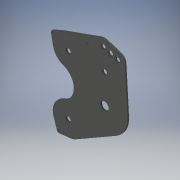
# Autodesk Inventor part: Shooter Side Plate
Saved by Autodesk Inventor 2019.4 (Build 234330000, 330)
## iProperties
Created: 2020-01-16
Part Number: Shooter Side Plate
Material: CFRP
Document SubType Name: Modeling
Designer: admin
Density: 1.43 g/cm^3
Appearance: Carbon Fiber
Mass: 572.525 g
Surface Area: 1689.26 cm^2
Volume: 400.367 cm^3
Author: admin
Autodesk Inventor part; units mm, degrees
ref_plane "YZ Plane" through (0, 0, 0) normal (1, 0, 0) x (0, 1, 0)
ref_plane "XZ Plane" through (0, 0, 0) normal (0, 1, 0) x (-1, 0, 0)
ref_plane "XY Plane" through (0, 0, 0) normal (0, 0, 1) x (1, 0, 0)
sketch "Sketch1" plane through (0, 0, 0) normal (0, 0, 1) x (1, 0, 0)
  arc A0 (88.7461, 5.2288) -> (44.314, -77.068) centre (0, 0) ccw construction
  circle A1 centre (0, 114.3) radius 50.8 construction
  circle A2 centre (-140.8057, 114.3) radius 50.8 construction
  circle A3 centre (-140.8057, -114.3) radius 50.8 construction
  line L0 (-140.8057, 114.3) -> (-140.8057, -114.3) construction
  line L1 (-140.8057, 0) -> (0, 0) construction
  circle A4 centre (-140.8057, -114.3) radius 9.5
  circle A5 centre (-140.8057, 114.3) radius 9.5
  circle A6 centre (0, 114.3) radius 9.5
  line L2 (0, 0) -> (0, 114.3) construction
  circle A7 centre (-4.9132, 197.2883) radius 9
  circle A8 centre (50.8994, 180.0301) radius 9
  line L3 (0, 114.3) -> (50.8994, 180.0301) construction
  line L4 (0, 114.3) -> (-4.9132, 197.2883) construction
  arc A9 (59.0234, 206.3028) -> (78.3518, 181.6476) centre (50.8994, 180.0301) ccw construction
  arc A10 (-14.1538, 223.1893) -> (3.2107, 223.561) centre (-4.9132, 197.2883) ccw construction
  line L5 (0, 0) -> (-490.9821, 0) construction
  line L6 (78.3518, 181.6476) -> (88.7461, 5.2288)
  line L7 (3.2107, 223.561) -> (59.0234, 206.3028)
  arc A11 (-160.967, 170.8112) -> (-160.2677, 57.5441) centre (-140.8057, 114.3) ccw
  arc A12 (-160.2677, -57.5441) -> (-110.8974, -166.3144) centre (-140.8057, -114.3) ccw
  line L8 (-160.967, 170.8112) -> (-14.1538, 223.1893)
  line L9 (-110.8974, -166.3144) -> (44.314, -77.068)
  arc A13 (-160.2677, -57.5441) -> (-160.2677, 57.5441) centre (-180, 0) ccw
  arc A14 (44.314, -77.068) -> (88.7461, 5.2288) centre (0, 0) ccw
  arc A15 (-160.2677, 57.5441) -> (-160.967, 170.8112) centre (-140.8057, 114.3) ccw construction
  arc A16 (-110.8974, -166.3144) -> (-160.2677, -57.5441) centre (-140.8057, -114.3) ccw construction
  circle A17 centre (0, 0) radius 16
  line L10 (-140.8057, -114.3) -> (0, 114.3) construction
  line L11 (-140.8057, 114.3) -> (-88.5835, 196.6353) construction
  circle A18 centre (22.9931, 188.6592) radius 22.86 construction
  circle A19 centre (-4.9132, 197.2883) radius 6.35 construction
  circle A20 centre (50.8994, 180.0301) radius 6.35 construction
  line L12 (-4.9132, 197.2883) -> (50.8994, 180.0301) construction
  arc A21 (3.2107, 223.561) -> (-14.1538, 223.1893) centre (-4.9132, 197.2883) ccw
  arc A22 (78.3518, 181.6476) -> (59.0234, 206.3028) centre (50.8994, 180.0301) ccw
  circle A23 centre (22.9931, 188.6592) radius 9.5
  line L13 (0, 114.3) -> (22.9931, 188.6592) construction
  line L14 (22.9931, 188.6592) -> (-140.8057, 114.3) construction
  circle A24 centre (-64.9132, 178.5367) radius 2.75
  circle A25 centre (64, 85.1942) radius 2.75
  dimension "d37" = 177.8
  dimension "d38" = 101.6
  dimension "d39" = 101.6
  dimension "d40" = 101.6
  dimension "d41" = 19
  dimension "d42" = 19
  dimension "d43" = 19
  dimension "d44" = 114.3
  dimension "d46" = 228.6
  dimension "d47" = 18
  dimension "d48" = 18
  dimension "d50" = 55
  dimension "d52" = 55
  dimension "d54" = 0
  dimension "d55" = 140.8057
  dimension "d58" = 120
  dimension "d59" = 120
  dimension "d60" = 180
  dimension "d61" = 32
  dimension "d64" = 268.485
  dimension "d67" = 97.5
  dimension "d77" = 45.72
  dimension "d78" = 12.7
  dimension "d79" = 12.7
  dimension "d80" = 19
  dimension "d81" = 77.833
  dimension "d82" = 179.887
  dimension "d90" = 5.5
  dimension "d91" = 25
  dimension "d92" = 60
  dimension "d93" = 5.5
  dimension "d94" = 20
  dimension "d95" = 64
  constraints: 30 end point, 26 centre point, 22 point on circle, 11 coincident, 11 tangent, 2 midpoint, 2 perpendicular, 2 point on line, 1 equal length, 1 horizontal
  measures "d37" diameter of A0
  measures "d38" diameter of A1
  measures "d39" diameter of A2
  measures "d40" diameter of A3
  measures "d41" diameter of A4
  measures "d42" diameter of A5
  measures "d43" diameter of A6
  measures "d44" distance of L1.end L2.end
  measures "d46" distance of L0.start L0.end
  measures "d47" diameter of A7
  measures "d48" diameter of A8
  measures "d50" diameter of A9
  measures "d52" diameter of A10
  measures "d54" distance between parallel lines of L1 L5
  measures "d55" distance from line of point (0, 0) L0
  measures "d58" diameter of A11
  measures "d59" diameter of A12
  measures "d60" distance of point (0, 0) A13.centre
  measures "d61" diameter of A17
  measures "d64" distance of L10.start L2.end
  measures "d67" distance of L11.start L11.end
  measures "d77" diameter of A18
  measures "d78" diameter of A19
  measures "d79" diameter of A20
  measures "d80" diameter of A23
  measures "d81" distance of L2.end L13.end
  measures "d82" distance of L13.end L11.start
  measures "d90" diameter of A24
  measures "d91" distance from line of L8 A24.centre
  measures "d92" horizontal distance of A10.centre A24.centre
  measures "d93" diameter of A25
  measures "d94" distance from line of L6 A25.centre
  measures "d95" horizontal distance of L1.end A25.centre
extrude "Extrusion1" add sketch "Sketch1" along normal blind 5
sketch "Sketch4" plane through (0, 0, 5) normal (0, 0, 1) x (1, 0, 0)
  circle A0 centre (0, 0) radius 16 projected
  circle A1 centre (22.9931, 188.6592) radius 9.5 projected
  circle A2 centre (0, 114.3) radius 9.5 projected
  circle A3 centre (-140.8057, 114.3) radius 9.5 projected
  circle A4 centre (-140.8057, -114.3) radius 9.5 projected
  circle A5 centre (50.8994, 180.0301) radius 9 projected
  circle A6 centre (-4.9132, 197.2883) radius 9 projected
  line L0 (88.7461, 5.2288) -> (78.3518, 181.6476) projected
  arc A7 (78.3518, 181.6476) -> (59.0234, 206.3028) centre (50.8994, 180.0301) ccw projected
  line L1 (59.0234, 206.3028) -> (3.2107, 223.561) projected
  arc A8 (3.2107, 223.561) -> (-14.1538, 223.1893) centre (-4.9132, 197.2883) ccw projected
  line L2 (-14.1538, 223.1893) -> (-160.967, 170.8112) projected
  arc A9 (-160.967, 170.8112) -> (-160.2677, 57.5441) centre (-140.8057, 114.3) ccw projected
  arc A10 (-160.2677, -57.5441) -> (-160.2677, 57.5441) centre (-180, 0) ccw projected
  arc A11 (-160.2677, -57.5441) -> (-110.8974, -166.3144) centre (-140.8057, -114.3) ccw projected
  line L3 (-110.8974, -166.3144) -> (44.314, -77.068) projected
  arc A12 (44.314, -77.068) -> (88.7461, 5.2288) centre (0, 0) ccw projected
  line L4 (-154.2466, 151.9742) -> (-7.4334, 204.3522)
  arc A13 (-2.6976, 204.4536) -> (-7.4334, 204.3522) centre (-4.9132, 197.2883) ccw
  line L5 (-2.6976, 204.4536) -> (53.1151, 187.1954)
  arc A14 (58.3865, 180.4712) -> (53.1151, 187.1954) centre (50.8994, 180.0301) ccw
  line L6 (58.3865, 180.4712) -> (68.7807, 4.0524)
  arc A15 (34.3446, -59.7299) -> (68.7807, 4.0524) centre (0, 0) ccw
  line L7 (34.3446, -59.7299) -> (-120.8669, -148.9763)
  arc A16 (-153.7803, -76.4627) -> (-120.8669, -148.9763) centre (-140.8057, -114.3) ccw
  arc A17 (-153.7803, -76.4627) -> (-153.7803, 76.4627) centre (-180, 0) ccw
  arc A18 (-154.2466, 151.9742) -> (-153.7803, 76.4627) centre (-140.8057, 114.3) ccw
  line L8 (-28.273, 196.9173) -> (-18.3857, 169.2037)
  line L9 (-18.3857, 169.2037) -> (58.7824, 173.7503)
  circle A19 centre (0, 114.3) radius 24.5
  circle A20 centre (-140.8057, 114.3) radius 29.5
  circle A21 centre (0, 0) radius 36
  circle A22 centre (-140.8057, -114.3) radius 29.5
  line L10 (-161.5522, -93.3278) -> (-168.604, -85.538)
  line L11 (-153.8938, -76.5018) -> (-145.9695, -85.2555)
  line L12 (-170.3057, -114.3) -> (-179.8595, -122.9486)
  line L13 (-162.6756, -134.0979) -> (-170.4598, -141.1446)
  line L14 (-140.8057, -143.8) -> (-132.157, -153.3538)
  line L15 (-121.0078, -136.1699) -> (-113.3352, -144.6456)
  line L16 (-133.6109, -66.1973) -> (-43.3302, -104.3928)
  line L17 (-108.1101, -36.9575) -> (-8.8951, -84.5927)
  dimension "d83" = 20
  dimension "d84" = 15
  dimension "d85" = 20
  dimension "d86" = 20
  dimension "d87" = 20
  constraints: 28 end point, 25 point on circle, 10 centre point, 5 point on line, 4 parallel, 3 perpendicular, 2 line through centre, 9 other
  measures "d83" distance between parallel lines of L2 L4
  measures "d84" radial gap between concentric circles of A2 A19
  measures "d85" radial gap between concentric circles of A3 A20
  measures "d86" radial gap between concentric circles of A0 A21
  measures "d87" radial gap between concentric circles of A4 A22
sketch "Sketch5" plane through (0, 0, 0) normal (0, 0, -1) x (-1, 0, 0)
  circle A0 centre (-48.7473, 204.2467) radius 2
  circle A1 centre (-10.5326, 216.0633) radius 2
  circle A2 centre (-35.4536, 161.2551) radius 2
  circle A3 centre (2.7611, 173.0717) radius 2
  point P0 (0, 0)
  constraints: 4 centre point, 8 other
extrude "Extrusion3" cut sketch "Sketch5" against normal through all
sketch "Sketch6" plane through (0, 0, 5) normal (0, 0, 1) x (1, 0, 0)
  circle A0 centre (-177.1645, -171.1708) radius 2.75
  circle A1 centre (-177.1645, -171.1708) radius 7.5
  circle A2 centre (-200.518, 145.7751) radius 2.75
  circle A3 centre (-200.518, 145.7751) radius 7.5
  arc A4 (-160.967, 170.8112) -> (-160.2677, 57.5441) centre (-140.8057, 114.3) ccw projected
  line L0 (-207.8765, 144.325) -> (-199.6735, 102.6992)
  line L1 (-203.4802, 152.6654) -> (-164.5031, 169.422)
  arc A5 (-160.2677, -57.5441) -> (-110.8974, -166.3144) centre (-140.8057, -114.3) ccw projected
  line L2 (-184.2783, -173.5463) -> (-197.7164, -133.3043)
  line L3 (-176.3349, -178.6248) -> (-134.1688, -173.9318)
  point P0 (0, 0)
  dimension "d100" = 5.5
  dimension "d101" = 15
  dimension "d102" = 5.5
  dimension "d103" = 15
  constraints: 10 tangent, 8 end point, 8 point on circle, 4 centre point, 2 coincident
  measures "d100" diameter of A0
  measures "d101" diameter of A1
  measures "d102" diameter of A2
  measures "d103" diameter of A3
extrude "Extrusion4" add sketch "Sketch6" against normal up to surface (5 mm away)
body "Solid1"
